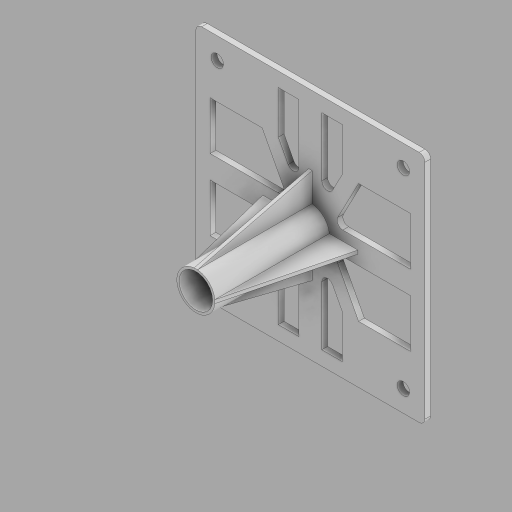
# Autodesk Inventor part: StiftHalter_PlateV1
Saved by Autodesk Inventor 2023 (Build 270158000, 158)
## iProperties
Created: 2024-02-15
Part Number: StiftHalter_PlateV1
Material: Generisch
Document SubType Name: Modeling
Designer: Nils Bade
Density: 1 g/cm^3
Appearance: Vorgabe
Description: Dummy
Auf Bestellliste: True
Author: Nils Bade
Autodesk Inventor part; units mm, degrees
ref_plane "YZ Plane" through (0, 0, 0) normal (1, 0, 0) x (0, 1, 0)
ref_plane "XZ Plane" through (0, 0, 0) normal (0, 1, 0) x (-1, 0, 0)
ref_plane "XY Plane" through (0, 0, 0) normal (0, 0, 1) x (1, 0, 0)
sketch "S-Basis" plane through (0, 0, 0) normal (0, 0, 1) x (1, 0, 0)
  line L0 (0, 57.19) -> (0, -57.19) construction
  line L1 (-56, 0) -> (56, 0) construction
  line L2 (-40, 40.85) -> (40, 40.85)
  line L3 (40, 40.85) -> (40, -40.85)
  line L4 (40, -40.85) -> (-40, -40.85)
  line L5 (-40, -40.85) -> (-40, 40.85)
  line L6 (-40, 40.85) -> (40, -40.85) construction
  line L7 (40, 40.85) -> (-40, -40.85) construction
  line L8 (-40, 33.35) -> (40, 33.35) construction
  circle A0 centre (-32.5, 33.35) radius 2.15
  circle A1 centre (32.5, 33.35) radius 2.15
  circle A2 centre (-32.5, -33.35) radius 2.15
  circle A3 centre (32.5, -33.35) radius 2.15
  line L9 (-4.418, 40.85) -> (4.418, 40.85)
  line L10 (-40, -40.85) -> (-16.2, -40.85) construction
  line L11 (-16.2, -40.85) -> (-16.2, -25.85) construction
  line L12 (-16.2, -25.85) -> (-40, -25.85) construction
  line L13 (-40, -25.85) -> (-40, -40.85) construction
  line L14 (-40, 40.85) -> (-16.2, 40.85) construction
  line L15 (-16.2, 40.85) -> (-16.2, 25.85) construction
  line L16 (-16.2, 25.85) -> (-40, 25.85) construction
  line L17 (-40, 25.85) -> (-40, 40.85) construction
  line L18 (40, -40.85) -> (16.2, -40.85) construction
  line L19 (16.2, -40.85) -> (16.2, -25.85) construction
  line L20 (16.2, -25.85) -> (40, -25.85) construction
  line L21 (40, -25.85) -> (40, -40.85) construction
  line L22 (40, 40.85) -> (16.2, 40.85) construction
  line L23 (40, 25.85) -> (40, 40.85) construction
  line L24 (16.2, 25.85) -> (40, 25.85) construction
  line L25 (16.2, 40.85) -> (16.2, 25.85) construction
  line L26 (-16.2, -35.85) -> (-14.2, -35.85)
  line L27 (-14.2, -35.85) -> (-14.2, -30.85)
  line L28 (-14.2, -30.85) -> (-16.2, -30.85)
  line L29 (-16.2, -30.85) -> (-16.2, -35.85)
  line L30 (-35, -25.85) -> (-30, -25.85)
  line L31 (-30, -25.85) -> (-30, -23.85)
  line L32 (-30, -23.85) -> (-35, -23.85)
  line L33 (-35, -23.85) -> (-35, -25.85)
  line L34 (-16.2, 35.85) -> (-14.2, 35.85)
  line L35 (-14.2, 35.85) -> (-14.2, 30.85)
  line L36 (-14.2, 30.85) -> (-16.2, 30.85)
  line L37 (-16.2, 30.85) -> (-16.2, 35.85)
  line L38 (-35, 25.85) -> (-30, 25.85)
  line L39 (-30, 25.85) -> (-30, 23.85)
  line L40 (-30, 23.85) -> (-35, 23.85)
  line L41 (-35, 23.85) -> (-35, 25.85)
  line L42 (16.2, -35.85) -> (14.2, -35.85)
  line L43 (14.2, -35.85) -> (14.2, -30.85)
  line L44 (14.2, -30.85) -> (16.2, -30.85)
  line L45 (16.2, -30.85) -> (16.2, -35.85)
  line L46 (35, -25.85) -> (30, -25.85)
  line L47 (30, -25.85) -> (30, -23.85)
  line L48 (30, -23.85) -> (35, -23.85)
  line L49 (35, -23.85) -> (35, -25.85)
  line L50 (14.2, 30.85) -> (16.2, 30.85)
  line L51 (14.2, 35.85) -> (14.2, 30.85)
  line L52 (16.2, 35.85) -> (14.2, 35.85)
  line L53 (16.2, 30.85) -> (16.2, 35.85)
  line L54 (30, 25.85) -> (30, 23.85)
  line L55 (30, 23.85) -> (35, 23.85)
  line L56 (35, 23.85) -> (35, 25.85)
  line L57 (35, 25.85) -> (30, 25.85)
  circle A4 centre (0, 0) radius 5.85
  circle A5 centre (0, 0) radius 6.65
  line L58 (0.6, 6.6229) -> (-0.6, 6.6229)
  line L59 (-0.6, 6.6229) -> (-0.6, 16.6229)
  line L60 (-0.6, 16.6229) -> (0.6, 16.6229)
  line L61 (0.6, 16.6229) -> (0.6, 6.6229)
  line L62 (-16.6229, -0.6) -> (-16.6229, 0.6)
  line L63 (-16.6229, 0.6) -> (-6.6229, 0.6)
  line L64 (-6.6229, -0.6) -> (-16.6229, -0.6)
  line L65 (-6.6229, 0.6) -> (-6.6229, -0.6)
  line L66 (0.6, -16.6229) -> (-0.6, -16.6229)
  line L67 (-0.6, -16.6229) -> (-0.6, -6.6229)
  line L68 (0.6, -6.6229) -> (0.6, -16.6229)
  line L69 (-0.6, -6.6229) -> (0.6, -6.6229)
  line L70 (16.6229, 0.6) -> (16.6229, -0.6)
  line L71 (16.6229, -0.6) -> (6.6229, -0.6)
  line L72 (6.6229, 0.6) -> (16.6229, 0.6)
  line L73 (6.6229, -0.6) -> (6.6229, 0.6)
  point P0 (0, 40.85)
  point P1 (-16.2, -33.35)
  point P2 (-16.2, 33.35)
  point P3 (16.2, -33.35)
  point P4 (16.2, 33.35)
  dimension "d0" = 81.7
  dimension "d1" = 80
  dimension "d4" = 7.5
  dimension "d7" = 4.3
  dimension "d8" = 32.5
  dimension "d9" = 4.3
  dimension "d10" = 32.5
  dimension "d11" = 7.5
  dimension "d26" = 15
  dimension "d27" = 23.8
  dimension "d30" = 5
  dimension "d31" = 5
  dimension "d32" = 5
  dimension "d33" = 2
  dimension "d34" = 2
  dimension "d85" = 11.7
  dimension "d86" = 0.8
  dimension "d87" = 1.2
  dimension "d88" = 10
  dimension "d91" = 360
  constraints: 144 end point, 38 symmetric about line, 10 parallel, 7 point on line, 6 centre point, 6 horizontal, 6 perpendicular, 5 midpoint, 2 point on circle, 1 coincident, 35 other
  measures "d0" distance of L2.end L3.end
  measures "d1" distance of L2.start L2.end
  measures "d4" distance between parallel lines of L8 L2
  measures "d7" diameter of A0
  measures "d8" distance from line of L0 A0.centre
  measures "d9" diameter of A2
  measures "d10" distance from line of L0 A2.centre
  measures "d11" distance from line of L4 A2.centre
  measures "d26" distance between parallel lines of L4 L12
  measures "d27" distance between parallel lines of L5 L11
  measures "d30" distance between parallel lines of L28 L26
  measures "d31" distance between parallel lines of L31 L33
  measures "d32" distance between parallel lines of L5 L33
  measures "d33" distance between parallel lines of L12 L32
  measures "d34" distance between parallel lines of L11 L27
  measures "d85" diameter of A4
  measures "d86" radial gap between concentric circles of A4 A5
  measures "d87" distance between parallel lines of L59 L61
  measures "d88" distance between parallel lines of L58 L60
extrude "Ex-Base1" add sketch "S-Basis" against normal blind 2 contours L2 L3 L4 L5 | L29 L28 L27 L26 | L33 L32 L31 L30 | L34 L35 L36 L37 | L38 L39 L40 L41 | L42 L43 L44 L45 | L46 L47 L48 L49 | L51 L52 L53 L50 | L57 L56 L55 L54 | A5 L73 | A5 L72 L70 L71 | L73 A5 L69 L65 L58 | L58 A5 | A5 L59 L60 L61 | L68 L66 L67 A5 | A5 L69 | L65 A5 | A5 L64 L62 L63
extrude "Ex-Probe" [suppressed]
fillet "Rundung1" radius 2 4 edges at (40, -40.85, -1) (-40, -40.85, -1) (40, 40.85, -1) (-40, 40.85, -1)
ref_plane "RWG-X" through (1.8795, 9, 10.525) normal (0, 0, -1) x (-1, 0, 0)
ref_plane "RWG-Y" through (0, 9, 9.585) normal (1, 0, 0) x (0, 0, -1)
sketch "Skizze5" plane through (0, 0, 0) normal (0, 0, 1) x (1, 0, 0)
  line L0 (0, 57.19) -> (0, -57.19) construction
  line L1 (-35, -4) -> (-35, -20.85)
  line L2 (-35, -20.85) -> (-16.8473, -20.85)
  line L3 (-16.8473, -20.85) -> (-8, -4)
  line L4 (-8, -4) -> (-35, -4)
  line L5 (-11.2, -20.85) -> (-11.2, -35.85)
  line L6 (-11.2, -35.85) -> (-4, -35.85)
  line L7 (-4, -35.85) -> (-4, -7.1374)
  line L8 (-4, -7.1374) -> (-11.2, -20.85)
  line L9 (-56, 0) -> (56, 0) construction
  line L10 (35, -4) -> (35, -20.85)
  line L11 (35, -20.85) -> (16.8473, -20.85)
  line L12 (16.8473, -20.85) -> (8, -4)
  line L13 (8, -4) -> (35, -4)
  line L14 (11.2, -20.85) -> (11.2, -35.85)
  line L15 (11.2, -35.85) -> (4, -35.85)
  line L16 (4, -35.85) -> (4, -7.1374)
  line L17 (4, -7.1374) -> (11.2, -20.85)
  point P0 (0, 0)
  dimension "d74" = 4
  dimension "d77" = 5
  dimension "d78" = 4
  constraints: 32 end point, 8 symmetric about line, 2 parallel, 2 perpendicular, 2 point on line, 2 vertical
  measures "d74" distance between parallel lines of L0 L7
  measures "d77" distance between parallel lines of L8 L3
  measures "d78" distance between parallel lines of L4 L9
extrude "Ex-ResinSave" cut sketch "Skizze5" against normal blind 2
fillet "Run-ResinSave" radius 2 4 edges at (-4, -7.1374, -1) (-8, -4, -1) (4, -7.1374, -1) (8, -4, -1)
mirror "Spiegeln3" about plane through (0, 0, 0) normal (0, 1, 0) of "Ex-ResinSave", "Run-ResinSave"
extrude "Ex-Führung" add sketch "S-Basis" along normal blind 40 contours A5 L73 | L73 A5 L69 L65 L58 | A5 L69
extrude "Ex-Stütze1" add sketch "S-Basis" along normal blind 40 contours L58 A5 | A5 L59 L60 L61
chamfer "Fase-Stütze1" distance 10 distance2 40 1 edges at (0, 16.6229, 40) measured on face at (0, 16.1229, 40)
pattern_circular "Runde Anordnung1" count 4 over 360 about axis through (0, 0, 0) along (0, 0, -1) of "Ex-Stütze1", "Fase-Stütze1"
equation "\"d10\" = d8"
equation "\"d11\" = d4"
